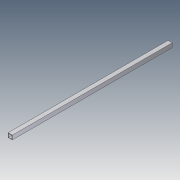
# Autodesk Inventor part: GE-12092-01
Saved by Autodesk Inventor 2012 (Build 160160000, 160)
## iProperties
Created: 2011-10-10
Part Number: GE-12092-01
Document SubType Name: Modeling
Designer: dfoster
Density: 1 g/cm^3
Description: Horizontal
Material: Default
Title: Horizontal
Author: dfoster
Autodesk Inventor part; units mm, degrees
ref_plane "YZ Plane" through (0, 0, 0) normal (1, 0, 0) x (0, 1, 0)
ref_plane "XZ Plane" through (0, 0, 0) normal (0, 1, 0) x (-1, 0, 0)
ref_plane "XY Plane" through (0, 0, 0) normal (0, 0, 1) x (1, 0, 0)
sketch "Sketch1" plane through (0, 0, 0) normal (0, 0, 1) x (1, 0, 0)
  line L0 (0, 0) -> (31.75, 0)
  line L1 (31.75, 0) -> (31.75, 31.75)
  line L2 (31.75, 31.75) -> (0, 31.75)
  line L3 (0, 31.75) -> (0, 0)
  line L4 (3.175, 28.575) -> (28.575, 28.575)
  line L5 (28.575, 28.575) -> (28.575, 3.175)
  line L6 (28.575, 3.175) -> (3.175, 3.175)
  line L7 (3.175, 3.175) -> (3.175, 28.575)
  dimension "d0" = 31.75
  dimension "d1" = 3.175
  constraints: 16 end point, 4 parallel, 3 perpendicular, 1 horizontal, 3 other
  measures "d0" distance of L1.end L2.end
  measures "d1" distance between parallel lines of L4 L2
extrude "Extrusion1" add sketch "Sketch1" along normal blind 1212.85
body "Solid1"
